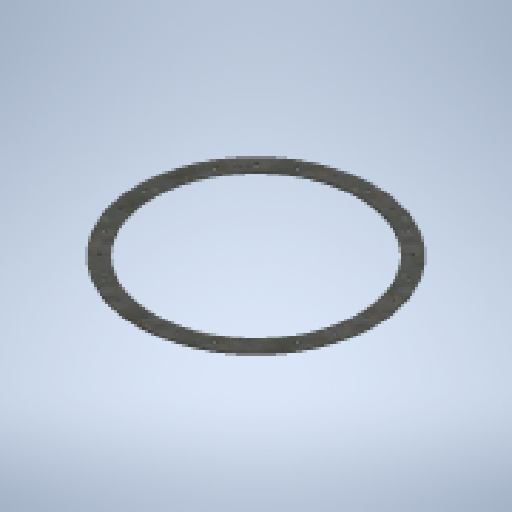
# Autodesk Inventor part: Tapa1
Saved by Autodesk Inventor 2023 (Build 270158000, 158)
## iProperties
RuleStatus: InUse
Created: 2022-11-02
Part Number: Tapa1
Material: Steel ASTM A36
Document SubType Name: Modeling
Designer: Juanse
Density: 7.85 g/cm^3
Appearance: Plate
Mass: 8991.62 g
Surface Area: 3341.83 cm^2
Volume: 1145.43 cm^3
Part_Area: 33418.255
Author: Juanse
Autodesk Inventor part; units mm, degrees
ref_plane "YZ Plane" through (0, 0, 0) normal (1, 0, 0) x (0, 1, 0)
ref_plane "XZ Plane" through (0, 0, 0) normal (0, 1, 0) x (-1, 0, 0)
ref_plane "XY Plane" through (0, 0, 0) normal (0, 0, 1) x (1, 0, 0)
sketch "Sketch1" plane through (0, 0, 0) normal (0, 1, 0) x (-1, 0, 0)
  circle A0 centre (0, 0) radius 420
  circle A1 centre (0, 0) radius 360
  circle A2 centre (390, 0) radius 7.1437
  circle A3 centre (0, 0) radius 390 construction
  dimension "d3" = 780
  dimension "d0" = 840
  dimension "d1" = 720
  dimension "d2" = 14.2875
  constraints: 3 centre point, 3 coincident, 2 horizontal alignment, 2 other
  measures "d0" diameter of A0
  measures "d1" diameter of A1
  measures "d2" diameter of A2
extrude "Extrusion1" add sketch "Sketch1" along normal blind 8 contours A0 | A2
hole "Hole1" at (-390, 0, 0) direction (0, 1, 0) diameter 14.2875 end through all
pattern_circular "Circular Pattern1" count 24 over 360 about axis through (0, 0, 0) along (0, 1, 0) of "Hole1"
equation "\"d6\" = d2"
equation "\"Part_Area\" = 33418.254582"
body "Solid1"
